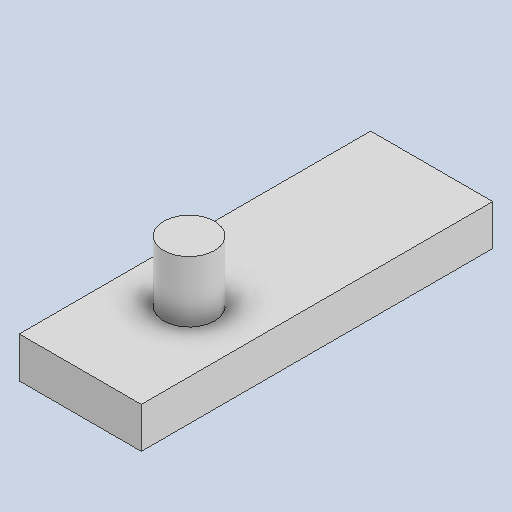
# Autodesk Inventor part: filler
Saved by Autodesk Inventor 2022 (Build 260153000, 153)
## iProperties
Created: 2022-02-25
Part Number: filler
Material: Generic
Document SubType Name: Modeling
Designer: Alexa
Density: 1 g/cm^3
Appearance: Default
Author: Alexa
Autodesk Inventor part; units mm, degrees
ref_plane "YZ Plane" through (0, 0, 0) normal (1, 0, 0) x (0, 1, 0)
ref_plane "XZ Plane" through (0, 0, 0) normal (0, 1, 0) x (-1, 0, 0)
ref_plane "XY Plane" through (0, 0, 0) normal (0, 0, 1) x (1, 0, 0)
sketch "Sketch6" plane through (0, 0, 0) normal (0, 1, 0) x (-1, 0, 0)
  line L0 (0, 0) -> (12, 0)
  line L1 (12, 0) -> (12, -34.549)
  line L2 (12, -34.549) -> (0, -34.549)
  line L3 (0, -34.549) -> (0, 0)
  dimension "d22" = 12
  dimension "d23" = 34.549
  constraints: 8 end point, 2 parallel, 1 horizontal, 1 perpendicular
  measures "d22" distance of L1.end L2.end
  measures "d23" distance of L0.end L1.end
extrude "Extrusion6" add sketch "Sketch6" along normal blind 4
sketch "Sketch7" plane through (0, 4, 0) normal (0, 1, 0) x (1, 0, 0)
  line L0 (-12, 0) -> (0, 0) projected
  line L1 (0, 0) -> (-6, 0)
  line L2 (-6, 0) -> (-6, 10.7)
  line L3 (-6, 10.7) -> (0, 10.7)
  line L4 (0, 10.7) -> (0, 0)
  circle A0 centre (-6, 10.7) radius 2.5
  dimension "d26" = 6
  dimension "d27" = 10.7
  dimension "d28" = 5
  constraints: 8 end point, 2 parallel, 1 centre point, 1 coincident, 1 horizontal, 1 perpendicular
  measures "d26" distance of L2.end L3.end
  measures "d27" distance of L1.end L2.end
  measures "d28" diameter of A0
extrude "Extrusion7" add sketch "Sketch7" along normal blind 6 contours A0 L3 L2 | L2 L3 A0
body "Solid2"
